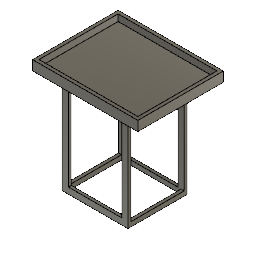
Projector Stand Drawing (Autodesk Fusion 360 archive; units mm, degrees)
design "skin"
Autodesk Fusion 360 part; units mm, degrees
sketch "Sketch1" plane through (0, 0, 0) normal (0, 0, 1) x (1, 0, 0)
  line L0 (50, -45) -> (-50, -45)
  line L1 (-50, -45) -> (-50, 45)
  line L2 (-50, 45) -> (50, 45)
  line L3 (50, 45) -> (50, -45)
  line L4 (50, -45) -> (-50, 45) construction
  line L5 (-50, -45) -> (50, 45) construction
  dimension "d35" = 90
  constraint perpendicular L0 L1
  constraint parallel L0 L2
  constraint parallel L1 L3
  constraint horizontal L0
  constraint coincident L4 origin
  constraint coincident L5 origin
  measures "d35" distance of L0.start L2.end
extrude "Extrude1" add sketch "Sketch1" along normal blind 150 makes body 1
sketch "Sketch2" plane through (0, 0, 150) normal (0, 0, 1) x (-1, 0, 0)
  line L0 (-50, -45) -> (50, -45)
  line L1 (50, -45) -> (50, 45)
  line L2 (50, 45) -> (-50, 45)
  line L3 (-50, 45) -> (-50, -45)
  line L4 (-45.0662, 40.4892) -> (45.0662, 40.4892)
  line L5 (45.0662, 40.4892) -> (45.0662, -40.4892)
  line L6 (45.0662, -40.4892) -> (-45.0662, -40.4892)
  line L7 (-45.0662, -40.4892) -> (-45.0662, 40.4892)
  line L8 (-45.0662, 40.4892) -> (45.0662, -40.4892) construction
  line L9 (45.0662, 40.4892) -> (-45.0662, -40.4892) construction
  constraint perpendicular L4 L5
  constraint parallel L4 L6
  constraint parallel L5 L7
  constraint horizontal L4
  constraint coincident L8 origin
  constraint coincident L9 origin
extrude "Extrude2" cut sketch "Sketch2" against normal blind 150 contours L4 L5 L6 L7 bodies 1
sketch "Sketch3" plane through (50, 0, 0) normal (1, 0, 0) x (0, 1, 0)
  line L0 (-45, 0) -> (45, 0)
  line L1 (45, 0) -> (45, 150)
  line L2 (45, 150) -> (-45, 150)
  line L3 (-45, 150) -> (-45, 0)
  line L4 (40.4892, 7.1838) -> (-40.4892, 7.1838)
  line L5 (-40.4892, 7.1838) -> (-40.4892, 142.8162)
  line L6 (-40.4892, 142.8162) -> (40.4892, 142.8162)
  line L7 (40.4892, 142.8162) -> (40.4892, 7.1838)
  line L8 (40.4892, 7.1838) -> (-40.4892, 142.8162) construction
  line L9 (-40.4892, 7.1838) -> (40.4892, 142.8162) construction
  line L10 (40.4892, 150) -> (40.4892, 0)
  point P0 (0, 75)
  constraint perpendicular L4 L5
  constraint parallel L4 L6
  constraint parallel L5 L7
  constraint horizontal L4
  constraint coincident L4.start L10
  constraint coincident L8 P0
  constraint coincident L9 P0
extrude "Extrude3" cut sketch "Sketch3" against normal blind 5 contours L4 L5 L6 L7 L10 bodies 1
sketch "Sketch4" plane through (0, -45, 0) normal (0, -1, 0) x (1, 0, 0)
  line L0 (-50, 0) -> (50, 0)
  line L1 (50, 0) -> (50, 150)
  line L2 (50, 150) -> (-50, 150)
  line L3 (-50, 150) -> (-50, 0)
  line L4 (40.45, 145.3077) -> (-40.45, 145.3077)
  line L5 (-40.45, 145.3077) -> (-40.45, 9.6577)
  line L6 (-40.45, 9.6577) -> (40.45, 9.6577)
  line L7 (40.45, 9.6577) -> (40.45, 145.3077)
  line L8 (40.45, 145.3077) -> (-40.45, 9.6577) construction
  line L9 (-40.45, 145.3077) -> (40.45, 9.6577) construction
  point P0 (0, 77.4827)
  dimension "d7" = 135.65
  dimension "d8" = 80.9
  constraint perpendicular L4 L5
  constraint parallel L4 L6
  constraint parallel L5 L7
  constraint horizontal L4
  constraint coincident L8 P0
  constraint coincident L9 P0
  measures "d7" distance of L4.end L5.end
  measures "d8" distance of L5.end L6.end
extrude "Extrude4" cut sketch "Sketch4" against normal blind 5 contours L4 L5 L6 L7 bodies 1
sketch "Sketch5" plane through (-50, 0, 0) normal (-1, 0, 0) x (0, -1, 0)
  line L0 (-45, 0) -> (45, 0)
  line L1 (45, 0) -> (45, 150)
  line L2 (45, 150) -> (-45, 150)
  line L3 (-45, 150) -> (-45, 0)
  line L4 (40.45, 7.185) -> (-40.45, 7.185)
  line L5 (-40.45, 7.185) -> (-40.45, 142.815)
  line L6 (-40.45, 142.815) -> (40.45, 142.815)
  line L7 (40.45, 142.815) -> (40.45, 7.185)
  line L8 (40.45, 7.185) -> (-40.45, 142.815) construction
  line L9 (-40.45, 7.185) -> (40.45, 142.815) construction
  point P0 (0, 75)
  dimension "d11" = 80.9
  dimension "d12" = 135.63
  constraint perpendicular L4 L5
  constraint parallel L4 L6
  constraint parallel L5 L7
  constraint horizontal L4
  constraint coincident L8 P0
  constraint coincident L9 P0
  measures "d11" distance of L5.end L6.end
  measures "d12" distance of L4.end L5.end
extrude "Extrude5" cut sketch "Sketch5" against normal blind 5 contours L4 L5 L6 L7 bodies 1
sketch "Sketch6" plane through (0, 45, 0) normal (0, 1, 0) x (-1, 0, 0)
  line L0 (-50, 0) -> (50, 0)
  line L1 (50, 0) -> (50, 150)
  line L2 (50, 150) -> (-50, 150)
  line L3 (-50, 150) -> (-50, 0)
  line L4 (40.45, 142.815) -> (-40.45, 142.815)
  line L5 (-40.45, 142.815) -> (-40.45, 7.185)
  line L6 (-40.45, 7.185) -> (40.45, 7.185)
  line L7 (40.45, 7.185) -> (40.45, 142.815)
  line L8 (40.45, 142.815) -> (-40.45, 7.185) construction
  line L9 (-40.45, 142.815) -> (40.45, 7.185) construction
  point P0 (0, 75)
  dimension "d15" = 135.63
  dimension "d16" = 80.9
  constraint perpendicular L4 L5
  constraint parallel L4 L6
  constraint parallel L5 L7
  constraint horizontal L4
  constraint coincident L8 P0
  constraint coincident L9 P0
  measures "d15" distance of L4.end L5.end
  measures "d16" distance of L5.end L6.end
extrude "Extrude6" cut sketch "Sketch6" against normal blind 5 contours L4 L5 L6 L7 bodies 1
sketch "Sketch7" plane through (0, 0, 0) normal (0, 0, 1) x (1, 0, 0)
sketch "Sketch8" plane through (0, 0, 0) normal (0, 0, 1) x (1, 0, 0)
  line L0 (80, -60, 150) -> (-80, -60, 150)
  line L1 (-80, -60, 150) -> (-80, 70, 150)
  line L2 (-80, 70, 150) -> (80, 70, 150)
  line L3 (80, 70, 150) -> (80, -60, 150)
  line L4 (80, -60, 150) -> (-80, 70, 150) construction
  line L5 (-80, -60, 150) -> (80, 70, 150) construction
  point P0 (0, 5)
extrude "Extrude7" add sketch "Sketch8" along normal blind 15 separate body contours L0 L1 L2 L3 in plane through (0, 0, 150) normal (0, 0, 1) makes body 2
sketch "Sketch9" plane through (0, 0, 0) normal (0, 1, 0) x (1, 0, 0)
sketch "Sketch10" plane through (0, 0, 0) normal (0, 0, 1) x (1, 0, 0)
  line L0 (75, -55, 165) -> (-75, -55, 165)
  line L1 (-75, -55, 165) -> (-75, 65, 165)
  line L2 (-75, 65, 165) -> (75, 65, 165)
  line L3 (75, 65, 165) -> (75, -55, 165)
  line L4 (75, -55, 165) -> (-75, 65, 165) construction
  line L5 (-75, -55, 165) -> (75, 65, 165) construction
  point P0 (0, 5)
extrude "Extrude8" cut sketch "Sketch10" against normal blind 10 contours L0 L1 L2 L3 in plane through (0, 0, 165) normal (0, 0, 1) bodies 1 2
extrude "Extrude9" cut 1 faces at (-46.7108, 13.4833, 142.815) along direction (0, 0, 1) blind 10 on bodies 1 bodies 1
extrude "Extrude10" cut 1 faces at (13.4833, -43.4964, 145.3077) along direction (0, 0, 1) blind 20 on bodies 1 bodies 1
extrude "Extrude11" cut 1 faces at (46.7108, -13.4964, 142.8162) along direction (0, 0, 1) blind 10 on bodies 1 bodies 1
extrude "Extrude12" cut 1 faces at (-13.4833, 43.4964, 142.815) along direction (0, 0, 1) blind 15 on bodies 1 bodies 1
equation "d35 = width"
equation "width = 90 mm"
